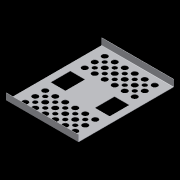
# Autodesk Inventor part: Belly Pan
Saved by Autodesk Inventor 2014 SP1 (Build 180222100, 222)
## iProperties
Created: 2013-11-29
Part Number: Belly Pan
Material: Aluminum 6061
Document SubType Name: Sheet Metal
Designer: Rauhul Varma
Mass: 3095.7 g
Surface Area: 7547.75 cm^2
Volume: 1142.32 cm^3
Density: 2.71 g/cm^3
Sheet Metal Rule: Default
Appearance: Aluminum - Flat
Flat Pattern Width: 55.88 cm
Flat Pattern Length: 83.9863 cm
Flat Pattern Area: 4693.16 cm^2
Sheet Metal Width: 22.000 in
Sheet Metal Length: 33.065 in
Sheet Metal Area: 727.441 in^2
Author: Rauhul Varma
Autodesk Inventor part; units mm, degrees
ref_plane "YZ Plane" through (0, 0, 0) normal (1, 0, 0) x (0, 1, 0)
ref_plane "XZ Plane" through (0, 0, 0) normal (0, 1, 0) x (-1, 0, 0)
ref_plane "XY Plane" through (0, 0, 0) normal (0, 0, 1) x (1, 0, 0)
sketch "Sketch2" plane through (0, 0, 0) normal (0, 1, 0) x (-1, 0, 0)
  line L0 (0, 0) -> (558.8, 0)
  line L1 (558.8, 0) -> (558.8, 736.6)
  line L2 (558.8, 736.6) -> (0, 736.6)
  line L3 (0, 736.6) -> (0, 0)
  line L4 (50.8, 736.6) -> (50.8, 0)
  line L5 (508, 736.6) -> (508, 0)
  line L6 (50.8, 698.5) -> (508, 698.5)
  line L7 (508, 38.1) -> (50.8, 38.1)
  line L8 (0, 368.3) -> (558.8, 368.3)
  line L9 (50.8, 444.5) -> (165.1, 444.5)
  line L10 (165.1, 444.5) -> (165.1, 292.1)
  line L11 (165.1, 292.1) -> (50.8, 292.1)
  line L12 (508, 292.1) -> (393.7, 292.1)
  line L13 (393.7, 292.1) -> (393.7, 444.5)
  line L14 (393.7, 444.5) -> (508, 444.5)
  line L15 (63.5, 698.5) -> (63.5, 457.2)
  line L16 (63.5, 457.2) -> (177.8, 457.2)
  line L17 (177.8, 457.2) -> (177.8, 279.4)
  line L18 (177.8, 279.4) -> (63.5, 279.4)
  line L19 (63.5, 279.4) -> (63.5, 38.1)
  line L20 (495.3, 698.5) -> (495.3, 457.2)
  line L21 (495.3, 457.2) -> (381, 457.2)
  line L22 (381, 457.2) -> (381, 279.4)
  line L23 (381, 279.4) -> (495.3, 279.4)
  line L24 (495.3, 279.4) -> (495.3, 38.1)
  circle A0 centre (85.725, 676.275) radius 22.225
  circle A1 centre (85.725, 598.805) radius 22.225
  circle A2 centre (85.725, 521.335) radius 22.225
  circle A3 centre (163.195, 676.275) radius 22.225
  circle A4 centre (163.195, 598.805) radius 22.225
  circle A5 centre (163.195, 521.335) radius 22.225
  circle A6 centre (240.665, 676.275) radius 22.225
  circle A7 centre (240.665, 598.805) radius 22.225
  circle A8 centre (240.665, 521.335) radius 22.225
  circle A9 centre (318.135, 676.275) radius 22.225
  circle A10 centre (318.135, 598.805) radius 22.225
  circle A11 centre (318.135, 521.335) radius 22.225
  circle A12 centre (395.605, 676.275) radius 22.225
  circle A13 centre (395.605, 598.805) radius 22.225
  circle A14 centre (395.605, 521.335) radius 22.225
  circle A15 centre (473.075, 676.275) radius 22.225
  circle A16 centre (473.075, 598.805) radius 22.225
  circle A17 centre (473.075, 521.335) radius 22.225
  circle A18 centre (85.725, 60.325) radius 22.225
  circle A19 centre (85.725, 137.795) radius 22.225
  circle A20 centre (85.725, 215.265) radius 22.225
  circle A21 centre (163.195, 60.325) radius 22.225
  circle A22 centre (163.195, 137.795) radius 22.225
  circle A23 centre (163.195, 215.265) radius 22.225
  circle A24 centre (240.665, 60.325) radius 22.225
  circle A25 centre (240.665, 137.795) radius 22.225
  circle A26 centre (240.665, 215.265) radius 22.225
  circle A27 centre (318.135, 60.325) radius 22.225
  circle A28 centre (318.135, 137.795) radius 22.225
  circle A29 centre (318.135, 215.265) radius 22.225
  circle A30 centre (395.605, 60.325) radius 22.225
  circle A31 centre (395.605, 137.795) radius 22.225
  circle A32 centre (395.605, 215.265) radius 22.225
  circle A33 centre (473.075, 60.325) radius 22.225
  circle A34 centre (473.075, 137.795) radius 22.225
  circle A35 centre (473.075, 215.265) radius 22.225
  line L25 (85.725, 676.275) -> (163.195, 598.805) construction
  line L26 (163.195, 676.275) -> (85.725, 598.805) construction
  circle A36 centre (124.46, 637.54) radius 17.4625
  circle A37 centre (124.46, 560.07) radius 17.4625
  circle A38 centre (201.93, 637.54) radius 17.4625
  circle A39 centre (201.93, 560.07) radius 17.4625
  circle A40 centre (279.4, 637.54) radius 17.4625
  circle A41 centre (279.4, 560.07) radius 17.4625
  circle A42 centre (356.87, 637.54) radius 17.4625
  circle A43 centre (356.87, 560.07) radius 17.4625
  circle A44 centre (434.34, 637.54) radius 17.4625
  circle A45 centre (434.34, 560.07) radius 17.4625
  line L27 (85.725, 60.325) -> (163.195, 137.795) construction
  line L28 (163.195, 60.325) -> (85.725, 137.795) construction
  circle A46 centre (124.46, 99.06) radius 17.4625
  circle A47 centre (124.46, 176.53) radius 17.4625
  circle A48 centre (201.93, 99.06) radius 17.4625
  circle A49 centre (201.93, 176.53) radius 17.4625
  circle A50 centre (279.4, 99.06) radius 17.4625
  circle A51 centre (279.4, 176.53) radius 17.4625
  circle A52 centre (356.87, 99.06) radius 17.4625
  circle A53 centre (356.87, 176.53) radius 17.4625
  circle A54 centre (434.34, 99.06) radius 17.4625
  circle A55 centre (434.34, 176.53) radius 17.4625
  dimension "d2" = 558.8
  dimension "d3" = 736.6
  dimension "d25" = 50.8
  dimension "d26" = 50.8
  dimension "d27" = 38.1
  dimension "d28" = 38.1
  dimension "d29" = 114.3
  dimension "d30" = 114.3
  dimension "d31" = 152.4
  dimension "d32" = 152.4
  dimension "d33" = 12.7
  dimension "d34" = 12.7
  dimension "d35" = 12.7
  dimension "d36" = 12.7
  dimension "d37" = 12.7
  dimension "d38" = 12.7
  dimension "d39" = 12.7
  dimension "d40" = 12.7
  dimension "d41" = 12.7
  dimension "d42" = 12.7
  dimension "d43" = 44.45
  dimension "d46" = 77.47
  dimension "d49" = 77.47
  dimension "d52" = 44.45
  dimension "d55" = 77.47
  dimension "d58" = 77.47
  dimension "d61" = 34.925
  dimension "d64" = 77.47
  dimension "d67" = 77.47
  dimension "d70" = 34.925
  dimension "d73" = 77.47
  dimension "d76" = 77.47
  constraints: 58 end point, 56 centre point, 16 point on line, 14 perpendicular, 8 parallel, 5 horizontal, 4 midpoint, 4 tangent, 4 vertical, 1 collinear, 106 other
  measures "d2" distance of L2.end L1.end
  measures "d3" distance of L1.end L0.end
  measures "d25" distance between parallel lines of L4 L3
  measures "d26" distance between parallel lines of L1 L5
  measures "d27" distance between parallel lines of L6 L2
  measures "d28" distance between parallel lines of L7 L0
  measures "d29" distance of L13.end L14.end
  measures "d30" distance of L9.start L9.end
  measures "d31" distance between parallel lines of L11 L9
  measures "d32" distance between parallel lines of L12 L14
  measures "d33" distance between parallel lines of L15 L4
  measures "d34" distance between parallel lines of L16 L9
  measures "d35" distance between parallel lines of L17 L10
  measures "d36" distance between parallel lines of L11 L18
  measures "d37" distance between parallel lines of L4 L19
  measures "d38" distance between parallel lines of L5 L20
  measures "d39" distance between parallel lines of L21 L14
  measures "d40" distance between parallel lines of L22 L13
  measures "d41" distance between parallel lines of L12 L23
  measures "d42" distance between parallel lines of L5 L24
  measures "d43" diameter of A0
  measures "d46" distance of L25.start L26.end
  measures "d49" distance of L25.start L26.start
  measures "d52" diameter of A18
  measures "d55" distance of L27.start L28.end
  measures "d58" distance of L27.start L28.start
  measures "d61" diameter of A36
  measures "d64" distance of A36.centre A37.centre
  measures "d67" distance of A36.centre A38.centre
  measures "d70" diameter of A46
  measures "d73" distance of A46.centre A47.centre
  measures "d76" distance of A46.centre A48.centre
extrude "Plate1" add sketch "Sketch2" along normal blind 3.175 contours L3 L8 L4 L0 | L4 L7 L5 L0 | L3 L2 L4 L8 | L5 L8 L1 L0 | L4 L11 L10 L8 L17 L18 L19 L7 | L8 L10 L11 L4 | L4 L9 L10 L8 | L7 L24 L23 L22 L8 L13 L12 L5 | L19 A18 L7 | L2 L5 L6 L4 | L4 L6 L15 L16 L17 L8 L10 L9 | L8 L5 L2 L1 | L12 L13 L8 L5 | L7 A33 L24 | A21 | A24 | A27 | A30 | A34 | A35 | A20 | A19 | A18 L19 L18 L17 L8 L22 L23 L24 A33 L7 | A18 | A17 | A16 | A12 | A9 | A6 | A3 | A1 | A2 | L17 L16 L15 A0 L6 A15 L20 L21 L22 L8 | L8 L13 L14 L5 | A33 | L5 L14 L13 L8 L22 L21 L20 L6 | L6 A0 L15 | L20 A15 L6 | A0 | A15 | A4 | A5 | A7 | A8 | A10 | A11 | A13 | A14 | A22 | A23 | A25 | A26 | A28 | A29 | A31 | A32 | A36 | A37 | A38 | A39 | A40 | A41 | A42 | A43 | A44 | A45 | A46 | A47 | A48 | A49 | A50 | A51 | A52 | A53 | A54 | A55
extrude "Cut2" cut sketch "Sketch2" along normal blind 3.175 contours L8 L10 L11 L4 | L4 L9 L10 L8 | L12 L13 L8 L5 | A21 | A24 | A27 | A30 | A34 | A35 | A20 | A19 | A18 | A17 | A16 | A12 | A9 | A6 | A3 | A1 | A2 | L8 L13 L14 L5 | A33 | A0 | A15 | A4 | A5 | A7 | A8 | A10 | A11 | A13 | A14 | A22 | A23 | A25 | A26 | A28 | A29 | A31 | A32 | A36 | A37 | A38 | A39 | A40 | A41 | A42 | A43 | A44 | A45 | A46 | A47 | A48 | A49 | A50 | A51 | A52 | A53 | A54 | A55
sketch "Sketch12" plane through (0, 3.175, 736.6) normal (0, 0, 1) x (1, 0, 0)
  line L0 (-558.8, 0) -> (0, 0)
  line L1 (0, 0) -> (0, 50.8)
  line L2 (0, 50.8) -> (-558.8, 50.8)
  line L3 (-558.8, 50.8) -> (-558.8, 0)
  constraints: 6 end point, 1 horizontal, 1 perpendicular, 1 vertical
edge flange "Flange5" height 50.8 angle 90 thickness 3.175 bend radius 3.175 thickness toward (0, 0, 1) relief straight relief width 3.175 relief depth 1.5875 corner gap 3.175 corner form 0 edges at (-279.4, 3.175, 736.6) (-279.4, 3.175, 0) wall of the first edge with corners at (-558.8, 3.175, 736.6) (0, 3.175, 736.6) (0, 53.975, 736.6) (-558.8, 53.975, 736.6)
bend "Bend9"
corner "Corner5"
equation "\"d46\" = d49"
equation "\"d55\" = d46"
equation "\"d58\" = d55"
equation "\"d64\" = d46"
equation "\"d67\" = d49"
equation "\"d73\" = d55"
equation "\"d76\" = d58"
equation "\"d83\" = Thickness"
equation "\"d146\" = BendReliefWidth"
equation "\"d147\" = BendReliefDepth"
equation "\"d148\" = MinimumRemnant"
equation "\"d149\" = BendRadius"
equation "\"d152\" = BendRadius"
equation "\"d153\" = CornerReliefSize"
equation "\"d154\" = GapSize"
equation "\"d155\" = JacobiRadiusSize"
equation "\"BendRadius\" = Thickness"
equation "\"BendReliefWidth\" = Thickness"
equation "\"BendReliefDepth\" = 0.5 * Thickness"
equation "\"CornerReliefSize\" = 4 * Thickness"
equation "\"MinimumRemnant\" = 2 * Thickness"
equation "\"TransitionRadius\" = BendRadius"
equation "\"JacobiRadiusSize\" = BendRadius"
equation "\"GapSize\" = Thickness"
equation "\"d4\" = BendRadius"
equation "\"root2\" = 1.414214"
equation "\"Thickness\" = 3.175"
body "Solid1"
